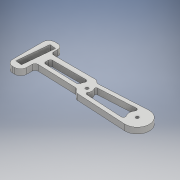
# Autodesk Inventor part: tipper_link_C
Saved by Autodesk Inventor 2017.2 (Build 212233000, 233)
## iProperties
Created: 2017-08-28
Part Number: tipper_link_C
Material: Generic
Document SubType Name: Modeling
Designer: Nic
Density: 1 g/cm^3
Appearance: Default
Author: Nic
Autodesk Inventor part; units mm, degrees
ref_plane "YZ Plane" through (0, 0, 0) normal (1, 0, 0) x (0, 1, 0)
ref_plane "XZ Plane" through (0, 0, 0) normal (0, 1, 0) x (-1, 0, 0)
ref_plane "XY Plane" through (0, 0, 0) normal (0, 0, 1) x (1, 0, 0)
sketch "Sketch1" plane through (0, 0, 0) normal (0, 0, 1) x (1, 0, 0)
  circle A0 centre (0, 0) radius 1.5
  arc A1 (-0.6702, -11.9813) -> (0, 12) centre (0, 0) ccw
  circle A2 centre (-50, 0) radius 1.5
  arc A3 (-6.6581, 4.4351) -> (-6.6581, -4.4351) centre (0, 0) ccw
  line L0 (-44.9603, 5.4977) -> (-8.4343, 7.5407)
  line L1 (-44.9603, -5.4977) -> (-8.4343, -7.5407)
  arc A4 (-44.9603, 5.4977) -> (-46.0589, 3.0769) centre (-44.8765, 4) ccw
  arc A5 (-46.0589, -3.0769) -> (-44.9603, -5.4977) centre (-44.8765, -4) ccw
  arc A6 (-6.6581, 4.4351) -> (-8.4343, 7.5407) centre (-8.3226, 5.5439) ccw
  arc A7 (-8.4343, -7.5407) -> (-6.6581, -4.4351) centre (-8.3226, -5.5439) ccw
  line L2 (-104, 0) -> (-57, 0) construction
  line L3 (-106, -18) -> (-104, -18)
  line L4 (-98, -12) -> (-98, -6.6741)
  line L5 (-112, -12) -> (-112, 18)
  arc A8 (-94.8953, -3.6759) -> (-98, -6.6741) centre (-95, -6.6741) ccw
  arc A9 (-106, 24) -> (-112, 18) centre (-106, 18) ccw
  arc A10 (-112, -12) -> (-106, -18) centre (-106, -12) ccw
  arc A11 (-104, -18) -> (-98, -12) centre (-104, -12) ccw
  arc A12 (-46.0589, -3.0769) -> (-46.0589, 3.0769) centre (-50, 0) ccw
  line L6 (-103, 19) -> (-106, -12) construction
  line L7 (-106.0856, 19.2986) -> (-109.0856, -11.7014)
  line L8 (-109.0856, -11.7014) -> (-102.9144, -12.2986)
  line L9 (-106.0856, 19.2986) -> (-99.9144, 18.7014)
  line L10 (-99.9144, 18.7014) -> (-102.9144, -12.2986)
  line L11 (-106, 24) -> (-103, 24)
  arc A13 (-98, 15) -> (-95, 12) centre (-95, 15) ccw
  line L12 (-95, 12) -> (-54, 12)
  line L13 (-47.8018, 9.3262) -> (0, 12)
  line L14 (-50.2234, -9.2095) -> (-0.6702, -11.9813)
  line L15 (-56.9088, -5.0024) -> (-94.8953, -3.6759)
  arc A14 (-51.0126, 10.66) -> (-54, 12) centre (-54, 8) ccw
  arc A15 (-51.0126, 10.66) -> (-47.8018, 9.3262) centre (-48.0252, 13.32) ccw
  arc A16 (-53.5242, -7.1079) -> (-50.2234, -9.2095) centre (-50, -5.2158) ccw
  arc A17 (-53.5242, -7.1079) -> (-56.9088, -5.0024) centre (-57.0484, -9) ccw
  line L16 (-91.3398, 7) -> (-58.0777, 7)
  line L17 (-59.5071, -0.9093) -> (-91.5071, 0.2082)
  line L18 (-93.4361, 2.2768) -> (-93.3386, 5.0698)
  arc A18 (-56.3772, 3.9474) -> (-57.4505, 0.8601) centre (-50, 0) ccw
  arc A19 (-59.5071, -0.9093) -> (-57.4505, 0.8601) centre (-59.4373, 1.0895) ccw
  arc A20 (-56.3772, 3.9474) -> (-58.0777, 7) centre (-58.0777, 5) ccw
  arc A21 (-91.3398, 7) -> (-93.3386, 5.0698) centre (-91.3398, 5) ccw
  arc A22 (-93.4361, 2.2768) -> (-91.5071, 0.2082) centre (-91.4373, 2.207) ccw
  line L19 (-98, 15) -> (-98, 19)
  arc A23 (-98, 19) -> (-103, 24) centre (-103, 19) ccw
  point P0 (-0.4468, -7.9875)
  point P1 (-94.8178, 5.6675)
  point P2 (-94.8178, 5.6675)
  point P3 (-52.6926, 7)
  point P4 (-57.4355, -0.9816)
  dimension "d0" = 3
  dimension "d2" = 12
  dimension "d10" = 50
  dimension "d14" = 16
  dimension "d18" = 2
  dimension "d31" = 7
  dimension "d42" = 3
  dimension "d43" = 6
  dimension "d52" = 14
  dimension "d53" = 98
  dimension "d57" = 18
  dimension "d60" = 24
  dimension "d61" = 3.1
  dimension "d63" = 5
  dimension "d77" = 8
  dimension "d80" = 4
  dimension "d81" = 4
  dimension "d82" = 4
  dimension "d83" = 4
  dimension "d84" = 1.5
  dimension "d85" = 9
  dimension "d86" = 4
  dimension "d87" = 8
  dimension "d88" = 178
  dimension "d90" = 5
  dimension "d91" = 4
  dimension "d92" = 7.5
  dimension "d93" = 2
  dimension "d94" = 2
  dimension "d95" = 32
  dimension "d96" = 5
  constraints: 47 point on circle, 40 end point, 37 tangent, 24 centre point, 8 equal radius, 6 coincident, 5 parallel, 4 horizontal, 4 vertical alignment, 3 point on line, 3 vertical, 2 concentric, 2 horizontal alignment, 2 midpoint, 2 perpendicular, 2 symmetric about line, 3 other
  measures "d0" diameter of A0
  measures "d2" radius of A1
  measures "d10" distance of point (0, 0) A2.centre
  measures "d14" diameter of A3
  measures "d18" radius of A6
  measures "d31" distance of A2.centre L2.end
  measures "d42" radius of A8
  measures "d43" radius of A9
  measures "d52" distance between parallel lines of L4 L5
  measures "d53" distance from line of point (0, 0) L4
  measures "d57" distance between parallel lines of L3 L2
  measures "d60" distance between parallel lines of L2 L11
  measures "d61" distance between parallel lines of L6 L10
  measures "d63" radius of A12
  measures "d77" distance of A5.centre A4.centre
  measures "d80" radius of A17
  measures "d81" radius of A16
  measures "d82" radius of A15
  measures "d83" radius of A14
  measures "d84" radius of A4
  measures "d85" vertical distance of A2.centre A17.centre
  measures "d86" horizontal distance of A2.centre A14.centre
  measures "d87" vertical distance of A12.centre A14.centre
  measures "d88" angle of L2 L15
  measures "d90" distance between parallel lines of L12 L16
  measures "d91" distance between parallel lines of L15 L17
  measures "d92" radius of A18
  measures "d93" radius of A19
  measures "d94" radius of A21
  measures "d95" horizontal distance of A19.centre A22.centre
  measures "d96" radius of A23
extrude "Extrusion1" add sketch "Sketch1" along normal blind 5.85
body "Solid1"
